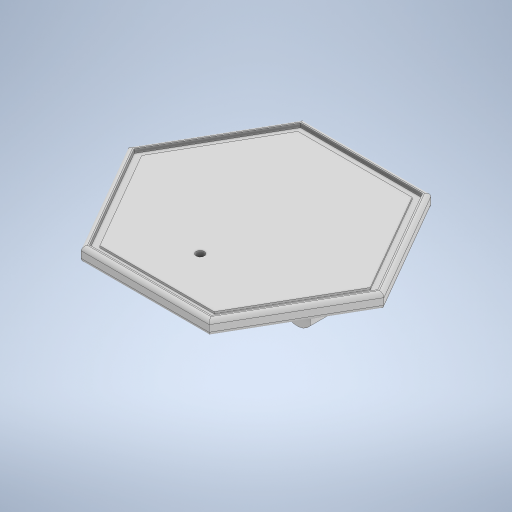
# Autodesk Inventor part: OV-PAM_n_6_bottom
Saved by Autodesk Inventor 2024 (Build 280153000, 153)
## iProperties
Created: 2023-08-31
Part Number: OV-PAM_n_6_bottom
Material: 일반
Document SubType Name: Modeling
Designer: jsw
Density: 1 g/cm^3
Appearance: 기본값
Author: jsw
Autodesk Inventor part; units mm, degrees
ref_plane "YZ Plane" through (0, 0, 0) normal (1, 0, 0) x (0, 1, 0)
ref_plane "XZ Plane" through (0, 0, 0) normal (0, 1, 0) x (-1, 0, 0)
ref_plane "XY Plane" through (0, 0, 0) normal (0, 0, 1) x (1, 0, 0)
sketch "스케치1" plane through (0, 0, 0) normal (0, 1, 0) x (-1, 0, 0)
  line L0 (17.6385, -30.5508) -> (-17.6385, -30.5508)
  line L1 (-17.6385, -30.5508) -> (-35.277, 0)
  line L2 (-35.277, 0) -> (-17.6385, 30.5508)
  line L3 (-17.6385, 30.5508) -> (17.6385, 30.5508)
  line L4 (17.6385, 30.5508) -> (35.277, 0)
  line L5 (35.277, 0) -> (17.6385, -30.5508)
  line L6 (19.486, -33.7508) -> (-19.486, -33.7508)
  line L7 (-19.486, -33.7508) -> (-38.972, 0)
  line L8 (-38.972, 0) -> (-19.486, 33.7508)
  line L9 (-19.486, 33.7508) -> (19.486, 33.7508)
  line L10 (19.486, 33.7508) -> (38.972, 0)
  line L11 (38.972, 0) -> (19.486, -33.7508)
  point P0 (0, 0)
  point P1 (0, 0)
  point P2 (0, 0)
  dimension "d0" = 70.554
  dimension "d1" = 3.2
  constraints: 24 end point, 2 coincident, 2 horizontal, 26 other
  measures "d0" distance of L2.end L0.start
  measures "d1" distance between parallel lines of L0 L6
extrude "돌출1" add sketch "스케치1" along normal blind 4.4 contours L0 L1 L2 L3 L4 L5 | L6 L7 L8 L9 L10 L11
sketch "스케치2" plane through (0, 4.4, 0) normal (0, 1, 0) x (1, 0, 0)
  line L0 (-18.5623, 32.1508) -> (18.5623, 32.1508)
  line L1 (18.5623, 32.1508) -> (37.1245, 0)
  line L2 (37.1245, 0) -> (18.5623, -32.1508)
  line L3 (18.5623, -32.1508) -> (-18.5623, -32.1508)
  line L4 (-18.5623, -32.1508) -> (-37.1245, 0)
  line L5 (-37.1245, 0) -> (-18.5623, 32.1508)
  line L6 (-19.486, 33.7508) -> (-38.972, 0) projected
  point P0 (0, 0)
  point P1 (0, 0)
  dimension "d4" = 1.6
  constraints: 12 end point, 1 coincident, 1 horizontal, 13 other
  measures "d4" distance between parallel lines of L5 L6
extrude "돌출2" cut sketch "스케치2" against normal blind 1.2
sketch "스케치3" plane through (0, 3.2, 0) normal (0, 1, 0) x (1, 0, 0)
  line L0 (17.4076, -30.1508) -> (-17.4076, -30.1508)
  line L1 (-17.4076, -30.1508) -> (-34.8151, 0)
  line L2 (-34.8151, 0) -> (-17.4076, 30.1508)
  line L3 (-17.4076, 30.1508) -> (17.4076, 30.1508)
  line L4 (17.4076, 30.1508) -> (34.8151, 0)
  line L5 (34.8151, 0) -> (17.4076, -30.1508)
  line L6 (-18.5623, 32.1508) -> (18.5623, 32.1508) projected
  point P0 (0, 0)
  point P1 (0, 0)
  dimension "d7" = 2
  constraints: 12 end point, 1 coincident, 1 horizontal, 13 other
  measures "d7" distance between parallel lines of L6 L3
extrude "돌출3" add sketch "스케치3" along normal blind 0.6
fillet "모깎기1" radius 1.2 12 edges at (0, 4.4, -33.7508) (0, 0, -33.7508) (-29.229, 4.4, -16.8754) (-29.229, 0, -16.8754) (-29.229, 4.4, 16.8754) (-29.229, 0, 16.8754) (0, 0, 33.7508) (0, 4.4, 33.7508) (29.229, 0, 16.8754) (29.229, 4.4, 16.8754) (29.229, 4.4, -16.8754) (29.229, 0, -16.8754)
sketch "스케치6" plane through (0, 0, 0) normal (0, -1, 0) x (1, 0, 0)
  line L0 (-20, -2.5) -> (-10, -2.5)
  line L1 (-10, -2.5) -> (-10, 2.5)
  line L2 (-10, 2.5) -> (-20, 2.5)
  line L3 (-20, 2.5) -> (-20, -2.5)
  line L4 (-20, -2.5) -> (-10, 2.5) construction
  line L5 (-10, -2.5) -> (-20, 2.5) construction
  line L6 (10, -2.5) -> (20, -2.5)
  line L7 (20, -2.5) -> (20, 2.5)
  line L8 (20, 2.5) -> (10, 2.5)
  line L9 (10, 2.5) -> (10, -2.5)
  line L10 (10, -2.5) -> (20, 2.5) construction
  line L11 (20, -2.5) -> (10, 2.5) construction
  point P0 (0, 0)
  point P1 (-15, 0)
  point P2 (15, 0)
  point P3 (-10, 0)
  point P4 (10, 0)
  dimension "d27" = 10
  dimension "d28" = 5
  dimension "d29" = 10
  dimension "d30" = 5
  dimension "d31" = 20
  dimension "d32" = 10
  constraints: 24 end point, 6 midpoint, 4 parallel, 2 horizontal, 2 horizontal alignment, 2 perpendicular
  measures "d27" distance of L2.end L1.end
  measures "d28" distance of L1.end L0.end
  measures "d29" distance of L8.end L7.end
  measures "d30" distance of L7.end L6.end
  measures "d31" distance of point (-10, 0) point (10, 0)
  measures "d32" distance of point (-10, 0) point (0, 0)
extrude "돌출6" add sketch "스케치6" along normal blind 10
sketch "스케치7" plane through (-10, 0, -2.5) normal (0, 0, -1) x (-1, 0, 0)
  line L0 (10, -10) -> (0, -10) projected
  circle A0 centre (5, -10) radius 5
  line L1 (-30, -10) -> (-20, -10) projected
  circle A1 centre (-25, -10) radius 5
  point P0 (-10, 0)
  constraints: 2 horizontal alignment, 2 midpoint, 4 other
extrude "돌출7" add sketch "스케치7" against normal blind 5
sketch "스케치8" plane through (-10, 0, -2.5) normal (0, 0, -1) x (-1, 0, 0)
  arc A0 (0, -10) -> (10, -10) centre (5, -10) ccw projected
  circle A1 centre (5, -10) radius 1.25
  arc A2 (-30, -10) -> (-20, -10) centre (-25, -10) ccw projected
  circle A3 centre (-25, -10) radius 1.25
  point P0 (-10, 0)
  dimension "d37" = 2.5
  dimension "d38" = 2.5
  constraints: 2 centre point, 2 coincident
  measures "d37" diameter of A1
  measures "d38" diameter of A3
extrude "돌출8" cut sketch "스케치8" against normal blind 5
sketch "스케치9" plane through (0, 0, 0) normal (0, -1, 0) x (1, 0, 0)
  line L0 (-20, 2.5) -> (-20, -2.5) projected
  line L1 (-10, -2.5) -> (-20, -2.5) projected
  line L2 (-10, -2.5) -> (-10, 2.5) projected
  line L3 (-20, 2.5) -> (-10, 2.5) projected
  line L4 (10, 2.5) -> (10, -2.5) projected
  line L5 (20, -2.5) -> (10, -2.5) projected
  line L6 (20, -2.5) -> (20, 2.5) projected
  line L7 (10, 2.5) -> (20, 2.5) projected
  line L8 (-19, 2.5) -> (-19, -2.5)
  line L9 (19, 2.5) -> (19, -2.5)
  point P0 (0, 0)
  dimension "d41" = 1
  dimension "d42" = 1
  constraints: 4 end point, 4 point on line, 2 perpendicular
  measures "d41" distance between parallel lines of L0 L8
  measures "d42" distance between parallel lines of L6 L9
extrude "돌출9" cut sketch "스케치9" along normal blind 15 contours L3 L8 L1 L0 | L7 L6 L5 L9
sketch "스케치10" plane through (0, 0, 0) normal (0, -1, 0) x (1, 0, 0)
  circle A0 centre (0, 17) radius 1.25
  point P0 (0, 0)
  dimension "d45" = 2.5
  dimension "d46" = 17
  constraints: 1 centre point, 1 vertical alignment
  measures "d45" diameter of A0
  measures "d46" distance of point (0, 0) A0.centre
extrude "돌출10" cut sketch "스케치10" against normal up to surface (3.8 mm away)
equation "\"d32\" = 0.5 * d31"
